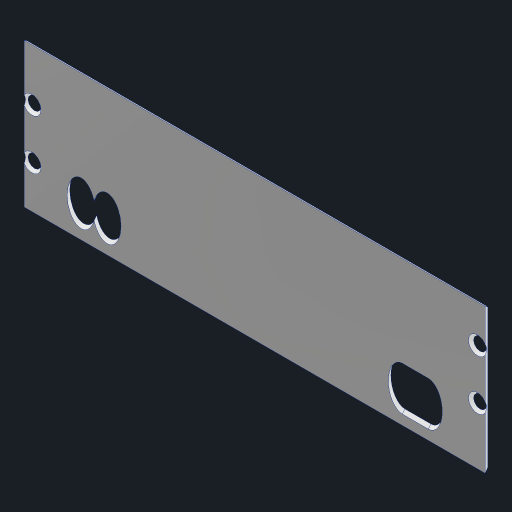
# Autodesk Inventor part: front
Saved by Autodesk Inventor 2023 (Build 270158000, 158)
## iProperties
Created: 2024-04-25
Part Number: front
Material: Aluminum 6061
Document SubType Name: Modeling
Designer: szymo
Density: 2.7 g/cm^3
Appearance: Aluminum - Flat
Mass: 36.9176 g
Surface Area: 195.912 cm^2
Volume: 13.6732 cm^3
Author: szymo
Autodesk Inventor part; units mm, degrees
ref_plane "Work Plane1" through (0, 4.7283, -22.9522) normal (-1, 0, 0) x (0, -0.8411785, 0.5407576)
sketch "Sketch1" plane through (0, 4.7283, -22.9522) normal (-1, 0, 0) x (0, -0.8411785, 0.5407576)
  line L0 (61.5, -12.25) -> (61.5, -16.75) projected
  line L1 (61.5, -16.75) -> (65.5, -16.75) projected
  line L2 (65.5, -16.75) -> (65.5, -20.25) projected
  line L3 (65.5, -20.25) -> (79.5, -20.25) projected
  line L4 (79.5, -20.25) -> (65.5, -11.25) projected
  line L5 (65.5, -11.25) -> (65.5, -12.25) projected
  line L6 (65.5, -12.25) -> (61.5, -12.25) projected
  line L7 (16.3889, 16.75) -> (16.3889, 18.75) projected
  line L8 (14.7421, 12.75) -> (16.3889, 18.75)
  line L9 (63.3493, -12.25) -> (12.0798, 20.7089)
  line L10 (16.3889, 16.75) -> (16.3889, 17.9388)
  arc A0 (-57.551, -16.75) -> (-61.5, -12.801) centre (-58.75, -14) ccw projected
  arc A1 (-34.301, -16.75) -> (-36.699, -16.75) centre (-35.5, -14) ccw projected
  line L11 (61.5, -12.25) -> (16.3889, 16.75) projected
  line L12 (16.3889, 13.75) -> (-61.5, 13.75) projected
  line L13 (-61.5, 13.75) -> (-61.5, -12.801) projected
  line L14 (-61.5, 13.75) -> (-61.5, -12.801) projected
  arc A2 (-57.551, -16.75) -> (-61.5, -12.801) centre (-58.75, -14) ccw projected
  line L15 (-57.551, -16.75) -> (-36.699, -16.75) projected
  arc A3 (-34.301, -16.75) -> (-36.699, -16.75) centre (-35.5, -14) ccw projected
  line L16 (-34.301, -16.75) -> (61.5, -16.75) projected
  line L17 (61.5, -16.75) -> (61.5, -12.25) projected
  line L18 (21.0556, 13.75) -> (-61.5, 13.75) projected
  line L19 (-57.551, -16.75) -> (-36.699, -16.75) projected
  line L20 (-34.301, -16.75) -> (61.5, -16.75) projected
  line L21 (61.5, -16.75) -> (61.5, -12.25) projected
  line L22 (61.5, -12.25) -> (21.0556, 13.75) projected
  point P0 (16.3889, 17.9388)
  point P1 (15.5655, 15.75)
  point P2 (16.3889, 17.9388)
  point P3 (16.1996, 18.0605)
  dimension "d14" = 1
  dimension "d15" = 2
  constraints: 6 end point, 3 point on line, 1 midpoint, 1 vertical
  measures "d14" distance between parallel lines of L9 L11
  measures "d15" distance from line of point (15.565, 15.75) L12
ref_plane "Work Plane2" through (178, -56.0619, -70.2985) normal (1, 0, 0) x (0, 0.8411785, -0.5407576)
extrude "Extrusion1" add sketch "Sketch1" against normal up to surface (178 mm away) contours L11 L7 L9 L6
sketch "Sketch2" plane through (0, -55.184, 1) normal (0, 0, 1) x (1, 0, 0)
  circle A0 centre (3, 16.4427) radius 2.5 projected
  circle A1 centre (3, 35.7569) radius 2.5 projected
  line L0 (0, 2.3333) -> (0, 55.184) projected
  line L1 (0, 2.3333) -> (3, 2.3333) projected
  line L2 (6, 50.414) -> (6, 9.4662) projected
  line L3 (0, 50.414) -> (6, 50.414) projected
  circle A2 centre (175, 21.9904) radius 2.5 projected
  circle A3 centre (175, 41.3047) radius 2.5 projected
  line L4 (178, 2.3333) -> (178, 55.9618) projected
  line L5 (178, 55.9618) -> (172, 55.9618) projected
  line L6 (172, 55.9618) -> (172, 2.3333) projected
  line L7 (178, 2.3333) -> (172, 2.3333) projected
  line L8 (3, 9.4662) -> (3, 2.3333) projected
  line L9 (3, 9.4662) -> (6, 9.4662) projected
  point P0 (3, 35.7569)
  point P1 (3, 16.4427)
  constraints: 4 coincident
hole "Hole1" at (3, -19.4271, 1) at (3, -38.7413, 1) at (175, -33.1936, 1) at (175, -13.8793, 1) direction (0, 0, -1) diameter 3.6 end through all countersink diameter 7 countersink angle 90 clearance for "Countersunk Flat Head Screw ISO 2009/7046" size "M3" standard "ISO"
ref_plane "Work Plane3" through (22, -31.0502, -8.6656) normal (0, -0.7712334, 0.6365525) x (1, 0, 0)
sketch "Sketch3" plane through (22, -31.0502, -8.6656) normal (0, -0.7712334, 0.6365525) x (1, 0, 0)
  line L0 (-9.9215, 5.3729) -> (-9.9215, -5.5323)
  spline S0 degree 3 poles (-9.9215, -5.5323) (-9.9222, -5.6561) (-9.8204, -5.8999) (-9.5772, -6.0011) (-9.4534, -6.0004) knots 0 0 0 0 0.5 1 1 1 1
  line L1 (-9.4534, -6.0004) -> (19.4534, -6.0004)
  spline S1 degree 3 poles (19.4534, -6.0004) (19.5775, -6.0011) (19.8219, -5.8989) (19.9222, -5.6548) (19.9215, -5.5307) knots 0 0 0 0 0.5 1 1 1 1
  line L2 (19.9215, -5.5307) -> (19.9215, 5.3744)
  spline S2 degree 3 poles (19.9215, 5.3744) (19.9222, 5.4985) (19.82, 5.743) (19.5758, 5.8433) (19.4518, 5.8426) knots 0 0 0 0 0.5 1 1 1 1
  line L3 (19.4518, 5.8426) -> (-9.4534, 5.8426)
  spline S3 degree 3 poles (-9.4534, 5.8426) (-9.5775, 5.8433) (-9.8219, 5.7411) (-9.9222, 5.4969) (-9.9215, 5.3729) knots 0 0 0 0 0.5 1 1 1 1
  circle A0 centre (-8.3791, -4.458) radius 0.5
  circle A1 centre (-8.3791, 4.3001) radius 0.5
  circle A2 centre (18.3791, 4.3001) radius 0.5
  circle A3 centre (18.3791, -4.458) radius 0.5
  arc A4 (5.2617, -1.5301) -> (5.1811, -1.6008) centre (5.2771, -1.6289) ccw
  arc A5 (5.1811, 1.4429) -> (5.1811, -1.6008) centre (0, -0.0789) ccw
  arc A6 (5.1811, 1.4429) -> (5.2617, 1.3723) centre (5.2771, 1.4711) ccw
  arc A7 (5.2617, 1.3723) -> (5.3414, 1.4401) centre (5.2463, 1.4711) ccw
  arc A8 (5.3414, -1.5979) -> (5.3414, 1.4401) centre (10, -0.0789) ccw
  arc A9 (5.3414, -1.5979) -> (5.2617, -1.5301) centre (5.2463, -1.6289) ccw
  line L4 (143.9215, 5.3729) -> (143.9215, -5.5323)
  spline S4 degree 3 poles (143.4534, 5.8426) (143.5775, 5.8433) (143.8219, 5.7411) (143.9222, 5.4969) (143.9215, 5.3729) knots 0 0 0 0 0.5 1 1 1 1
  line L5 (114.5482, 5.8426) -> (143.4534, 5.8426)
  spline S5 degree 3 poles (114.0785, 5.3744) (114.0778, 5.4985) (114.18, 5.743) (114.4242, 5.8433) (114.5482, 5.8426) knots 0 0 0 0 0.5 1 1 1 1
  line L6 (114.0785, -5.5307) -> (114.0785, 5.3744)
  spline S6 degree 3 poles (114.5466, -6.0004) (114.4225, -6.0011) (114.1781, -5.8989) (114.0778, -5.6548) (114.0785, -5.5307) knots 0 0 0 0 0.5 1 1 1 1
  line L7 (143.4534, -6.0004) -> (114.5466, -6.0004)
  spline S7 degree 3 poles (143.9215, -5.5323) (143.9222, -5.6561) (143.8204, -5.8999) (143.5772, -6.0011) (143.4534, -6.0004) knots 0 0 0 0 0.5 1 1 1 1
  circle A10 centre (142.3791, -4.458) radius 0.5
  circle A11 centre (142.3791, 4.3001) radius 0.5
  circle A12 centre (115.6209, 4.3001) radius 0.5
  circle A13 centre (115.6209, -4.458) radius 0.5
  arc A14 (128.8189, -1.6008) -> (128.7383, -1.5301) centre (128.7229, -1.6289) ccw
  arc A15 (128.7383, -1.5301) -> (128.6586, -1.5979) centre (128.7537, -1.6289) ccw
  arc A16 (128.6586, 1.4401) -> (128.6586, -1.5979) centre (124, -0.0789) ccw
  arc A17 (128.6586, 1.4401) -> (128.7383, 1.3723) centre (128.7537, 1.4711) ccw
  arc A18 (128.7383, 1.3723) -> (128.8189, 1.4429) centre (128.7229, 1.4711) ccw
  arc A19 (128.8189, -1.6008) -> (128.8189, 1.4429) centre (134, -0.0789) ccw
  circle A20 centre (10, -0.0789) radius 5.4
  circle A21 centre (124, -0.0789) radius 5.4
  line L8 (0, 5.3211) -> (10, 5.3211)
  line L9 (10, -5.4789) -> (0, -5.4789)
  line L10 (124, 5.3211) -> (134, 5.3211)
  line L11 (134, -5.4789) -> (124, -5.4789)
  point P0 (-22, 26.4483)
  point P1 (14.6373, -1.6617)
  point P2 (5, 1.9607)
  point P3 (5.3627, -1.6617)
  point P4 (5, -2.1185)
  point P5 (7.5029, -4.2949)
  point P6 (3.3743, -4.2949)
  point P7 (5.2923, -1.5401)
  dimension "d9" = 10.8
  dimension "d10" = 10.8
  constraints: 8 end point, 8 point on circle, 4 point on line, 3 tangent, 2 centre point, 2 coincident
  measures "d9" diameter of A20
  measures "d10" diameter of A21
extrude "Extrusion2" cut sketch "Sketch3" along normal blind 78.25 contours A9 A8 A7 A6 A5 A20 A4 | A4 A5 A20 A6 A7 A8 A9 | A5 A20 | A19 A21 A18 A17 A16 A15 A14 | A14 A15 A16 A17 A18 A19 A21 | A21 A19 | A19 L11 A21 | A19 A21 L10
body "Solid1"
